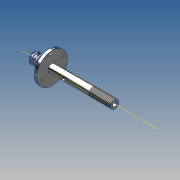
# Autodesk Inventor part: Einspritzdüse_ra8846s
Saved by Autodesk Inventor 2021 (Build 250183000, 183)
## iProperties
Created: 2020-12-19
Part Number: Einspritzdüse_ra8846s
Material: Aluminium 6061
Document SubType Name: Modeling
Designer: Ricardo
Density: 2.7 g/cm^3
Appearance: Aluminium - flach
Project: Motor
Mass: 0.667111 g
Surface Area: 6.67166 cm^2
Volume: 0.247078 cm^3
Author: Sander
Revision Number: Rev00
Autodesk Inventor part; units mm, degrees
ref_plane "YZ-Ebene" through (0, 0, 0) normal (1, 0, 0) x (0, 1, 0)
ref_plane "XZ-Ebene" through (0, 0, 0) normal (0, 1, 0) x (-1, 0, 0)
ref_plane "XY-Ebene" through (0, 0, 0) normal (0, 0, 1) x (1, 0, 0)
sketch "Skizze1" plane through (0, 0, 0) normal (0, 0, 1) x (1, 0, 0)
  line L0 (-35.4, 0) -> (5.9, 0) projected
  line L1 (0, -1.1) -> (0, 6.6) projected
  line L2 (0, 0.7) -> (-19.5, 0.7)
  line L3 (-19.5, 0.7) -> (-19.5, 1)
  line L4 (-19.5, 1) -> (-29.5, 1)
  line L5 (-29.5, 1) -> (-29.5, 1.5)
  line L6 (-29.5, 1.5) -> (-23.5, 1.5)
  line L7 (-23.5, 1.5) -> (-23.5, 5.5)
  line L8 (-23.5, 5.5) -> (-22.5, 5.5)
  line L9 (-22.5, 5.5) -> (-22.5, 1.5)
  line L10 (-22.5, 1.5) -> (0, 1.5)
  point P0 (0, 0)
  dimension "d0" = 1.4
  dimension "d1" = 3
  dimension "d2" = 10
  dimension "d3" = 22.5
  dimension "d4" = 1
  dimension "d5" = 6
  dimension "d6" = 2
  dimension "d7" = 11
  constraints: 18 end point, 7 perpendicular, 4 point on line, 1 horizontal
  measures "d0" diameter of L2.start L0
  measures "d1" diameter of L10.end L0
  measures "d2" distance of L3.end L4.end
  measures "d3" distance of L9.end L10.end
  measures "d4" distance of L7.end L8.end
  measures "d5" distance of L5.end L6.end
  measures "d6" diameter of L4.end L0
  measures "d7" diameter of L7.end L0
revolve "Umdrehung1" add sketch "Skizze1" angle 360 about axis through (-10, 0, 0) along (1, 0, 0)
sketch "Skizze2" plane through (0, 0, 0) normal (0, 0, 1) x (1, 0, 0)
  line L0 (-29.5, 1.5) -> (-23.5, 1.5) projected
  line L1 (-19.5, 1) -> (-29.5, 1) projected
  line L2 (-29.7, 1.5) -> (-29.7, 1)
  line L3 (-29.7, 1) -> (-29.5, 1)
  line L4 (-29.5, 1) -> (-27.7, 1)
  line L5 (-27.7, 1) -> (-27.7, 1.5)
  line L6 (-27.7, 1.5) -> (-28.0942, 1.5)
  line L7 (-28.0942, 1.5) -> (-28.2, 2.1)
  line L8 (-28.2, 2.1) -> (-29.0242, 1.8)
  line L9 (-29.0242, 1.8) -> (-29.1974, 1.5)
  line L10 (-29.1974, 1.5) -> (-29.7, 1.5)
  line L11 (-35.64, 0) -> (5.94, 0) projected
  point P0 (0, 0)
  dimension "d9" = 0.2
  dimension "d10" = 2
  dimension "d11" = 1.5
  dimension "d12" = 0.3
  dimension "d13" = 0.3
  dimension "d14" = 60
  dimension "d15" = 20
  dimension "d16" = 100
  constraints: 18 end point, 4 point on line, 2 collinear, 1 perpendicular, 1 vertical
  measures "d9" distance of L2.end L1.end
  measures "d10" distance of L4.end L2.end
  measures "d11" horizontal distance of L7.end L2.start
  measures "d12" vertical distance of L2.start L8.end
  measures "d13" vertical distance of L7.end L8.end
  measures "d14" angle of L0 L9
  measures "d15" angle of L0 L8
  measures "d16" angle of L0 L7
revolve "Umdrehung2" add sketch "Skizze2" angle 360 about axis through (-10, 0, 0) along (1, 0, 0) contours L9 L8 L7 L0
fillet "Rundung1" radius 0.2 3 edges at (-29.5, -1.5, 0) (-29.0242, -1.8, 0) (-28.2, -2.1, 0)
pattern_linear "Rechteckige Anordnung1" count 3 spacing 1.6 along (1, 0, 0) of "Umdrehung2"
fillet "Rundung2" radius 0.2 4 edges at (-27.4242, -1.8, 0) (-26.6, -2.1, 0) (-25.8242, -1.8, 0) (-25, -2.1, 0)
sketch "Skizze3" plane through (0, 0, 0) normal (0, 1, 0) x (-1, 0, 0)
  line L0 (35.4, 0) -> (-5.9, 0) projected
  line L1 (0, 0.7) -> (19.5, 0.7) projected
  line L2 (0, -0.7) -> (19.5, -0.7) projected
  line L3 (22.5, 5.5) -> (22.5, -5.5) projected
  circle A0 centre (17, 0) radius 0.5
  point P0 (0, 0)
  dimension "d23" = 1
  dimension "d24" = 5.5
  constraints: 1 centre point, 1 point on line
  measures "d23" diameter of A0
  measures "d24" distance from line of L3 A0.centre
extrude "Extrusion1" cut sketch "Skizze3" against normal through all both and the other way through all
thread "Gewinde1" size "M3x0.5" class "6g" standard "ANSI Metric M Profile" length 8
